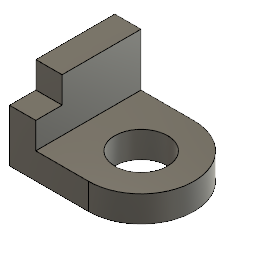
3DD4 (Autodesk Fusion 360 design; units mm, degrees)
Autodesk Fusion 360 part; units mm, degrees
sketch "Sketch1" plane through (0, 0, 0) normal (0, 1, 0) x (1, 0, 0)
  circle A0 centre (0, 0) radius 20
  circle A1 centre (0, 0) radius 10
  line L0 (-30, 20) -> (-30, -20)
  line L1 (-30, -20) -> (-20, -20)
  line L2 (0, 20) -> (-20, 20)
  line L3 (0, -20) -> (-20, -20)
  line L4 (-20, 20) -> (-30, 20)
  line L5 (-20, 20) -> (-20, -20)
  dimension "d1" = 40
  dimension "d2" = 20
  dimension "d3" = 40
  dimension "d4" = 10
  measures "d1" diameter of A0
  measures "d2" diameter of A1
extrude "Extrude1" add sketch "Sketch1" along normal blind 10
sketch "Sketch2" plane through (0, 10, 0) normal (0, 1, 0) x (-1, 0, 0)
  circle A0 centre (0, 0) radius 10
  arc A1 (0, 20) -> (0, -20) centre (0, 0) ccw
  line L0 (0, -20) -> (30, -20)
  line L1 (30, -20) -> (30, 20)
  line L2 (30, 20) -> (0, 20)
  line L3 (30, -20) -> (20, -20)
  line L4 (20, -20) -> (20, 20)
  line L5 (20, 20) -> (30, 20)
  line L6 (30, 20) -> (30, -20)
  dimension "d7" = 10
  dimension "d8" = 40
  measures "d8" distance of A0.centre
extrude "Extrude2" add sketch "Sketch2" along normal blind 20 contours L0 L1 L2 L3 L4 L5 L6
sketch "Sketch3" plane through (-20, 0, 0) normal (1, 0, 0) x (0, 0, -1)
  line L0 (-20, 10) -> (20, 10)
  line L1 (20, 10) -> (20, 30)
  line L2 (20, 30) -> (-20, 30)
  line L3 (-20, 30) -> (-20, 10)
  line L4 (-20, 30) -> (-10, 30)
  line L5 (-10, 30) -> (-10, 20)
  line L6 (-10, 20) -> (-20, 20)
  line L7 (-20, 20) -> (-20, 30)
  dimension "d11" = 10
  dimension "d12" = 10
  measures "d11" distance of origin
extrude "Extrude3" cut sketch "Sketch3" against normal blind 10 contours L2 L3 L4 L5 L6 L7
